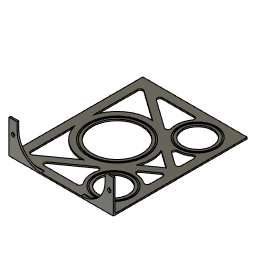
shelf-backer (Autodesk Fusion 360 design; units mm, degrees)
Autodesk Fusion 360 part; units mm, degrees
sketch "Sketch1" plane through (0, 0, 0) normal (0, 0, 1) x (1, 0, 0)
  line L0 (-74.0678, 23.5735) -> (-61.5678, 23.5735)
  line L1 (-61.5678, 23.5735) -> (-61.5678, 226.7735)
  line L2 (-61.5678, 226.7735) -> (-74.0678, 226.7735)
  line L3 (-74.0678, 226.7735) -> (-74.0678, 23.5735)
  line L4 (71.9322, 23.5735) -> (84.4322, 23.5735)
  line L5 (84.4322, 23.5735) -> (84.4322, 226.7735)
  line L6 (84.4322, 226.7735) -> (71.9322, 226.7735)
  line L7 (71.9322, 226.7735) -> (71.9322, 23.5735)
  line L8 (-32, 23.5735) -> (47, 23.5735) construction
  circle A0 centre (-67.8178, 5.0413) radius 2.55 construction
  circle A1 centre (78.1822, 4.9635) radius 2.55 construction
  line L9 (-74.0678, 26.0735) -> (-61.5678, 26.0735)
  line L10 (-61.5678, 26.0735) -> (-61.5678, 23.5735)
  line L11 (-61.5678, 23.5735) -> (-74.0678, 23.5735)
  line L12 (-74.0678, 23.5735) -> (-74.0678, 26.0735)
  line L13 (71.9322, 26.0735) -> (84.4322, 26.0735)
  line L14 (84.4322, 26.0735) -> (84.4322, 23.5735)
  line L15 (84.4322, 23.5735) -> (71.9322, 23.5735)
  line L16 (71.9322, 23.5735) -> (71.9322, 26.0735)
  line L17 (55.3253, 131.4235) -> (71.9322, 131.4235) construction
  line L18 (71.9322, 131.4235) -> (71.9322, 118.9235) construction
  line L19 (71.9322, 118.9235) -> (55.3253, 118.9235) construction
  line L20 (55.3253, 118.9235) -> (55.3253, 131.4235) construction
  line L21 (-61.5678, 23.5735) -> (71.9322, 118.9235)
  line L22 (71.9322, 131.4235) -> (-61.5678, 36.0735)
  line L23 (71.9322, 131.4235) -> (-61.5678, 226.7735)
  line L24 (71.9322, 118.9235) -> (-61.5678, 214.2735)
  line L25 (-61.5678, 23.5735) -> (71.9322, 23.5735)
  line L26 (67.9766, 35.4311) -> (-44.9659, 35.4311)
  circle A2 centre (46.9322, 61.3246) radius 22.5
  circle A3 centre (46.9322, 61.3246) radius 32.817
  circle A4 centre (-11.5678, 125.1735) radius 37.5
  circle A5 centre (-11.5678, 125.1735) radius 51.943
  line L27 (-61.5678, 226.7735) -> (71.9322, 226.7735)
  line L28 (71.9322, 214.2735) -> (-44.0665, 214.2735)
  line L29 (84.4322, 125.1735) -> (-74.0678, 125.1735) construction
  circle A6 centre (46.9322, 189.0223) radius 32.817
  circle A7 centre (46.9322, 189.0223) radius 22.5
  point P0 (-67.8178, 23.5735)
  point P1 (78.1822, 23.5735)
  point P2 (71.9322, 125.1735)
  point P3 (71.9322, 125.1735)
  dimension "d1" = 12.5
  dimension "d2" = 12.5
  dimension "d3" = 5.1
  dimension "d4" = 5.1
  dimension "d7" = 146
  dimension "d8" = 203.2
  dimension "d9" = 2.5
  dimension "d10" = 2.5
  dimension "d16" = 12.5
  dimension "d17" = 12.5
  dimension "d18" = 12.5
  dimension "d19" = 12.5
  dimension "d20" = 10.317
  dimension "d21" = 14.443
  dimension "d24" = 12.5
  dimension "d27" = 45
  dimension "d28" = 25
  dimension "d29" = 50
  dimension "d30" = 75
  constraint horizontal L0
  constraint vertical L1
  constraint horizontal L2
  constraint vertical L3
  constraint horizontal L4
  constraint vertical L5
  constraint horizontal L6
  constraint vertical L7
  constraint perpendicular L3 L8
  constraint coincident L4.start L8
  constraint coincident L0.end L8
  constraint midpoint L0 P0
  constraint vertical A0.centre P0
  constraint midpoint L4 P1
  constraint vertical A1.centre P1
  constraint equal L3 L5
  constraint horizontal L9
  constraint vertical L10
  constraint horizontal L11
  constraint vertical L12
  constraint coincident L3 L9.start
  constraint horizontal L13
  constraint vertical L14
  constraint horizontal L15
  constraint vertical L16
  constraint coincident L7 L13.start
  constraint horizontal L17
  constraint vertical L18
  constraint horizontal L19
  constraint vertical L20
  constraint midpoint L7 P3
  constraint midpoint L18 P3
  constraint horizontal P3 P2
  constraint coincident P3 P2
  constraint coincident L1 L22.end
  constraint coincident L1 L24.end
  constraint coincident L21 L26.end
  constraint parallel L25 L26
  constraint coincident L7 L28.start
  constraint coincident L23 L28.end
  constraint perpendicular L7 L28
  constraint midpoint L5 L29.start
  constraint midpoint L3 L29.end
  constraint symmetric A2 L29 A7
  constraint symmetric A3 L29 A6
  measures "d1" distance of L0.start L0.end
  measures "d2" distance of L4.start L4.end
  measures "d3" diameter of A0
  measures "d4" diameter of A1
  measures "d7" distance of L3 L7
  measures "d8" distance of L0.start L2.end
  measures "d9" distance of L0.end L9.end
  measures "d10" distance of L13.start L4.start
  measures "d16" distance of L17.start L19.end
  measures "d17" distance of L0.end L22.end
  measures "d18" distance of L1.end L24.end
  measures "d19" distance of L4.start L26.start
  measures "d24" distance of L27 L28
  measures "d27" diameter of A2
  measures "d28" distance of L7 A2.centre
  measures "d29" distance of L1 A4.centre
  measures "d30" diameter of A4
extrude "Extrude1" add sketch "Sketch1" along normal blind 50.8 contours L0 L1 L3 L9 L10 L11 L12 | L4 L5 L7 L13 L14 L15 L16 makes body 1 at (-69.9011, 26.0735, 16.9333) makes body 2 at (76.0989, 23.5735, 16.9333)
ref_plane "WorkPlane1" through (5.1822, 24.8235, 25.4) normal (1, 0, 0) x (0, 1, 0)
sketch "Sketch2" plane through (0, 23.5735, 0) normal (0, -1, 0) x (1, 0, 0)
  line L0 (-74.0678, 0) -> (-61.5678, 0)
  line L1 (-61.5678, 0) -> (-61.5678, 50.8)
  line L2 (-61.5678, 50.8) -> (-74.0678, 50.8)
  line L3 (-74.0678, 50.8) -> (-74.0678, 0)
  circle A0 centre (-67.8178, 30.5) radius 2.55
  line L4 (-74.0678, 0) -> (-61.5678, 0)
  line L5 (5.1822, 55.88) -> (5.1822, -5.08)
  circle A1 centre (78.1822, 30.5) radius 2.55
  line L6 (-69.5607, 32.3613) -> (-67.79, 34.0194)
  line L7 (-67.79, 34.0194) -> (-66.0457, 32.3336)
  line L8 (79.9252, 32.3613) -> (78.1545, 34.0194)
  line L9 (78.1545, 34.0194) -> (76.4101, 32.3336)
  point P0 (-67.8178, 50.8)
  dimension "d13" = 5.1
  dimension "d14" = 30.5
  constraint midpoint L2 P0
  constraint vertical A0.centre P0
  constraint symmetric A0 L5 A1
  constraint coincident A0 L6.start
  constraint coincident A0 L7.end
  constraint tangent A0 L7
  constraint tangent A0 L6
  constraint symmetric L5 L6.start L8.start
  constraint symmetric L5 L6.end L8.end
  constraint symmetric L5 L7.end L9.end
  measures "d13" diameter of A0
  measures "d14" distance of A0.centre L4
extrude "Extrude2" cut sketch "Sketch2" against normal through all contours A0 | A0 L6 L7 | A1 | A1 L8 L9 bodies 1 2
extrude "Extrude3" add sketch "Sketch1" along normal blind 2 contours L1 L10 L21 L22 L24 A3 A5 | L7 L16 L21 L25 L26 A3 | L1 L2 L3 L9 A5 | L21 A3 | L7 L21 L26 A3 | L26 A3 | L5 L6 L7 L13 A3 A6 | L1 L22 L23 L24 A5 A6 | L7 L23 L27 L28 A6 | L1 A5 | L1 L22 L24 A5 | L22 A5 | L7 A3 | L7 L22 L24 | L24 A5 | L7 L23 L28 A6 | L23 A6 | L28 A6 | L7 L28 A6 | L7 A6 bodies 1 2
fillet "Fillet2" radius 4 14 edges at (-61.5678, 36.0735, 1) (23.6038, 84.4057, 1) (26.7709, 35.4311, 1) (32.6668, 90.8788, 1) (71.9322, 118.9235, 1) (71.9322, 131.4235, 1) (32.6668, 159.4681, 1) (71.9322, 167.7631, 1) (-44.0665, 214.2735, 1) (23.6038, 165.9412, 1) (25.972, 214.2735, 1) (-61.5678, 214.2735, 1) (71.9322, 82.5838, 1) (-44.9659, 35.4311, 1) on bodies 1
sketch "Sketch3" plane through (0, 0, 2) normal (0, 0, 1) x (-1, 0, 0)
  line L0 (61.5678, -23.5735) -> (-71.9322, -23.5735)
  line L1 (-84.4322, -26.0735) -> (-84.4322, -226.7735)
  line L2 (-84.4322, -226.7735) -> (74.0678, -226.7735)
  line L3 (74.0678, -226.7735) -> (74.0678, -26.0735)
  line L4 (-36.8514, -143.9793) -> (-63.1816, -125.1735)
  line L5 (-63.1816, -125.1735) -> (-36.8514, -106.3676)
  arc A0 (-36.8514, -106.3676) -> (-36.8514, -143.9793) centre (11.5678, -125.1735) ccw
  line L6 (-47.2589, -101.301) -> (-65.6074, -114.4061)
  arc A1 (-71.9322, -111.151) -> (-65.6074, -114.4061) centre (-67.9322, -111.151) ccw
  line L7 (-71.9322, -111.151) -> (-71.9322, -91.5651)
  arc A2 (-65.6507, -88.2796) -> (-71.9322, -91.5651) centre (-67.9322, -91.5651) ccw
  arc A3 (-65.6507, -88.2796) -> (-49.2957, -94.0564) centre (-46.9322, -61.3246) ccw
  arc A4 (-47.2589, -101.301) -> (-49.2957, -94.0564) centre (-49.5838, -98.046) ccw
  circle A5 centre (11.5678, -125.1735) radius 37.5
  circle A6 centre (-46.9322, -189.0223) radius 22.5
  line L8 (55.2429, -209.7561) -> (9.4856, -177.0747)
  arc A7 (9.4856, -177.0747) -> (61.5678, -139.2473) centre (11.5678, -125.1735) ccw
  line L9 (61.5678, -139.2473) -> (61.5678, -206.501)
  arc A8 (55.2429, -209.7561) -> (61.5678, -206.501) centre (57.5678, -206.501) ccw
  circle A9 centre (-46.9322, -61.3246) radius 22.5
  arc A10 (-49.2957, -156.2905) -> (-65.6507, -162.0673) centre (-46.9322, -189.0223) ccw
  arc A11 (-71.9322, -158.7818) -> (-65.6507, -162.0673) centre (-67.9322, -158.7818) ccw
  line L10 (-71.9322, -158.7818) -> (-71.9322, -139.1959)
  arc A12 (-65.6074, -135.9409) -> (-71.9322, -139.1959) centre (-67.9322, -139.1959) ccw
  line L11 (-65.6074, -135.9409) -> (-47.2589, -149.0459)
  arc A13 (-49.2957, -156.2905) -> (-47.2589, -149.0459) centre (-49.5838, -152.3009) ccw
  line L12 (34.8081, -42.6861) -> (-9.0117, -73.9836)
  arc A14 (-15.2038, -69.7068) -> (-9.0117, -73.9836) centre (-11.3365, -70.7285) ccw
  arc A15 (-15.2038, -69.7068) -> (-20.5481, -41.8097) centre (-46.9322, -61.3246) ccw
  arc A16 (-17.3322, -35.4311) -> (-20.5481, -41.8097) centre (-17.3322, -39.4311) ccw
  line L13 (-17.3322, -35.4311) -> (32.4832, -35.4311)
  arc A17 (34.8081, -42.6861) -> (32.4832, -35.4311) centre (32.4832, -39.4311) ccw
  line L14 (61.5678, -43.8459) -> (61.5678, -111.0996)
  arc A18 (61.5678, -111.0996) -> (9.4856, -73.2722) centre (11.5678, -125.1735) ccw
  line L15 (9.4856, -73.2722) -> (55.2429, -40.5909)
  arc A19 (61.5678, -43.8459) -> (55.2429, -40.5909) centre (57.5678, -43.8459) ccw
  line L16 (31.5838, -214.2735) -> (-16.8677, -214.2735)
  arc A20 (-20.1341, -207.9646) -> (-16.8677, -214.2735) centre (-16.8677, -210.2735) ccw
  arc A21 (-20.1341, -207.9646) -> (-15.2038, -180.6401) centre (-46.9322, -189.0223) ccw
  arc A22 (-9.0117, -176.3633) -> (-15.2038, -180.6401) centre (-11.3365, -179.6184) ccw
  line L17 (-9.0117, -176.3633) -> (33.9087, -207.0184)
  arc A23 (31.5838, -214.2735) -> (33.9087, -207.0184) centre (31.5838, -210.2735) ccw
  circle A24 centre (-46.9322, -61.3246) radius 26.5
  circle A25 centre (-46.9322, -61.3246) radius 28.5
  circle A26 centre (11.5678, -125.1735) radius 41.5
  circle A27 centre (11.5678, -125.1735) radius 43.5
  circle A28 centre (-46.9322, -189.0223) radius 26.5
  circle A29 centre (-46.9322, -189.0223) radius 28.5
  line L18 (74.0678, -26.0735) -> (61.5678, -26.0735)
  line L19 (61.5678, -26.0735) -> (61.5678, -23.5735)
  line L20 (-71.9322, -23.5735) -> (-71.9322, -26.0735)
  line L21 (-71.9322, -26.0735) -> (-84.4322, -26.0735)
  dimension "d31" = 4
  dimension "d32" = 6
  dimension "d33" = 4
  dimension "d34" = 6
  dimension "d35" = 4
  dimension "d36" = 6
extrude "Extrude4" cut sketch "Sketch3" against normal blind 0.5 contours A25 | A27 | A29 bodies 1
fillet "Fillet3" radius 36.5 2 edges at (-61.5678, 24.8235, 2) (71.9322, 24.8235, 2) on bodies 1
fillet "Fillet4" radius 2.5 2 edges at (59.9322, 26.0735, 2) (-49.5678, 26.0735, 2) on bodies 1
